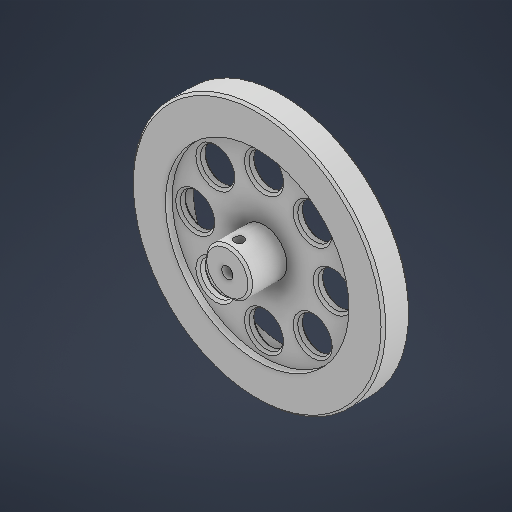
# Autodesk Inventor part: Flywheel
Saved by Autodesk Inventor 2025.4 (Build 294407000, 407)
## iProperties
Created: 2026-05-29
Part Number: Flywheel
Material: Generic
Document SubType Name: Modeling
Designer: VuQuan
Density: 1 g/cm^3
Appearance: Default
Author: VuQuan
Autodesk Inventor part; units mm, degrees
ref_plane "YZ Plane" through (0, 0, 0) normal (1, 0, 0) x (0, 1, 0)
ref_plane "XZ Plane" through (0, 0, 0) normal (0, 1, 0) x (-1, 0, 0)
sketch "Sketch1" plane through (0, 0, 0) normal (0, 0, 1) x (1, 0, 0)
  circle A0 centre (0, 0) radius 55
  circle A1 centre (0, 0) radius 40
  dimension "d0" = 110
  dimension "d1" = 80
  constraints: 2 centre point, 2 coincident
  measures "d0" diameter of A0
  measures "d1" diameter of A1
extrude "Extrusion1" add sketch "Sketch1" along normal blind 12
ref_plane "Work Plane1" through (0, 0, 5) normal (0, 0, -1) x (-1, 0, 0)
sketch "Sketch2" plane through (0, 0, 5) normal (0, 0, -1) x (-1, 0, 0)
  circle A0 centre (0, 0) radius 40 projected
  circle A1 centre (0, 30) radius 7.5
  circle A2 centre (0, 0) radius 10
  circle A3 centre (0, 0) radius 2.5
  dimension "d5" = 15
  dimension "d6" = 30
  dimension "d11" = 20
  dimension "d12" = 5
  constraints: 3 centre point, 2 coincident, 1 vertical alignment
  measures "d5" diameter of A1
  measures "d6" distance of point (0, 0) A1.centre
  measures "d11" diameter of A2
  measures "d12" diameter of A3
extrude "Extrusion2" add sketch "Sketch2" against normal blind 4 contours A0 | A1
extrude "Extrusion4" cut sketch "Sketch2" against normal blind 4 contours A1
extrude "Extrusion3" add sketch "Sketch2" against normal blind 20 contours A2
sketch "Sketch3" plane through (0, 0, 0) normal (0, 1, 0) x (-1, 0, 0)
  line L0 (10, 25) -> (-10, 25) projected
  line L1 (-10, 9) -> (10, 9) projected
  point P0 (0, 0)
  point P1 (0, 20)
  point P2 (0, 25)
  dimension "d17" = 5
  constraints: 1 midpoint, 1 vertical alignment
  measures "d17" distance from line of L0 point (0, 20)
hole "Hole1" at (0, 0, 20) direction (0, 1, 0) diameter 4.134 end through all thread size "M5x0.8" class "6H" standard "ISO Metric profile"
chamfer "Chamfer1" distance 1 angle 45 3 edges at (-55, 0, 12) (-55, 0, 0) (10, 0, 25)
chamfer "Chamfer2" distance 1 angle 45 2 edges at (7.5, 30, 5) (7.5, 30, 9)
pattern_circular "Circular Pattern1" count 8 over 360 about axis through (0, 0, 5) along (0, 0, 1) of "Extrusion4", "Chamfer2"
body "Solid1"
